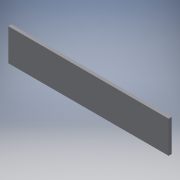
# Autodesk Inventor part: back_plate
Saved by Autodesk Inventor 2019 (Build 230136000, 136)
## iProperties
Created: 2021-11-19
Part Number: back_plate
Material: Generic
Document SubType Name: Modeling
Designer: Pokick
Density: 1 g/cm^3
Appearance: Default
Author: Pokick
Autodesk Inventor part; units mm, degrees
ref_plane "YZ Plane" through (0, 0, 0) normal (1, 0, 0) x (0, 1, 0)
ref_plane "XZ Plane" through (0, 0, 0) normal (0, 1, 0) x (-1, 0, 0)
ref_plane "XY Plane" through (0, 0, 0) normal (0, 0, 1) x (1, 0, 0)
sketch "Sketch1" plane through (0, 0, 0) normal (0, 0, 1) x (1, 0, 0)
  line L0 (0, 0) -> (-5.5, 0) construction
  line L1 (244.5, 50) -> (-255.5, 50)
  line L2 (-255.5, 50) -> (-255.5, -50)
  line L3 (-255.5, -50) -> (244.5, -50)
  line L4 (244.5, -50) -> (244.5, 50)
  line L5 (244.5, 50) -> (-255.5, -50) construction
  line L6 (-255.5, 50) -> (244.5, -50) construction
  dimension "d0" = 5.5
  dimension "d1" = 500
  dimension "d2" = 100
  constraints: 14 end point, 2 horizontal, 2 midpoint, 2 parallel, 1 perpendicular
  measures "d0" distance of L0.start L0.end
  measures "d1" distance of L3.end L2.end
  measures "d2" distance of L2.end L1.end
extrude "Extrusion1" add sketch "Sketch1" along normal blind 10
body "Solid1"
